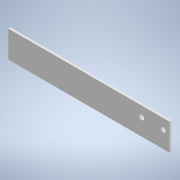
# Autodesk Inventor part: Part11
Saved by Autodesk Inventor 2020.2 (Build 242310000, 310)
## iProperties
Created: 2022-11-15
Part Number: Part11
Material: 一般
Document SubType Name: Modeling
Designer: Administrator
Density: 1 g/cm^3
Appearance: 既定
Author: Administrator
Autodesk Inventor part; units mm, degrees
ref_plane "YZ Plane" through (0, 0, 0) normal (1, 0, 0) x (0, 1, 0)
ref_plane "XZ Plane" through (0, 0, 0) normal (0, 1, 0) x (-1, 0, 0)
ref_plane "XY Plane" through (0, 0, 0) normal (0, 0, 1) x (1, 0, 0)
sketch "スケッチ1" plane through (0, 0, 0) normal (0, 0, 1) x (1, 0, 0)
  circle A0 centre (10, -9.3398) radius 2.25 projected
  circle A1 centre (-10, -9.3398) radius 2.25 projected
  line L0 (16, -14.3398) -> (16, 14.6602) projected
  line L1 (16, 14.6602) -> (4.899, 14.6602) projected
  arc A2 (-4.899, 14.6602) -> (4.899, 14.6602) centre (0, 15.6602) ccw projected
  line L2 (-4.899, 14.6602) -> (-16, 14.6602) projected
  line L3 (-16, 14.6602) -> (-16, -14.3398) projected
  line L4 (-16, -14.3398) -> (16, -14.3398) projected
  line L5 (16, 0.1602) -> (-134, 0.1602)
  line L6 (-134, 0.1602) -> (-134, -24.8398)
  line L7 (-134, -24.8398) -> (16, -24.8398)
  line L8 (16, -24.8398) -> (16, 0.1602)
  point P0 (0, 0)
  dimension "d0" = 150
  dimension "d1" = 25
  constraints: 8 end point, 2 parallel, 1 horizontal, 1 midpoint, 1 perpendicular
  measures "d0" distance of L7.end L6.end
  measures "d1" distance of L6.end L5.end
extrude "押し出し1" add sketch "スケッチ1" along normal blind 2 contours L4 L3 L5 L0 | L8 L7 L6 L5 L3 L4
